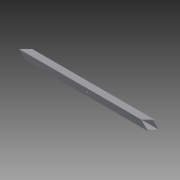
# Autodesk Inventor part: 1x1 support horizontal
Saved by Autodesk Inventor 2015 (Build 190159000, 159)
## iProperties
Created: 2015-01-22
Part Number: 1x1 support horizontal
Material: Generic
Document SubType Name: Modeling
Designer: 215152
Density: 1 g/cm^3
Appearance: Default
Author: 215152
Autodesk Inventor part; units mm, degrees
ref_plane "YZ Plane" through (0, 0, 0) normal (1, 0, 0) x (0, 1, 0)
ref_plane "XZ Plane" through (0, 0, 0) normal (0, 1, 0) x (-1, 0, 0)
ref_plane "XY Plane" through (0, 0, 0) normal (0, 0, 1) x (1, 0, 0)
sketch "Sketch1" plane through (0, 0, 0) normal (1, 0, 0) x (0, 1, 0)
  line L0 (0, 0) -> (-25.4, 0)
  line L1 (-25.4, 0) -> (-25.4, 25.4)
  line L2 (-25.4, 25.4) -> (0, 25.4)
  line L3 (0, 25.4) -> (0, 0)
  line L4 (-3.175, 3.175) -> (-22.225, 3.175)
  line L5 (-22.225, 3.175) -> (-22.225, 22.225)
  line L6 (-22.225, 22.225) -> (-3.175, 22.225)
  line L7 (-3.175, 22.225) -> (-3.175, 3.175)
  dimension "d0" = 25.4
  dimension "d1" = 25.4
  dimension "d2" = 19.05
  dimension "d3" = 19.05
  dimension "d4" = 3.175
  dimension "d5" = 3.175
  constraints: 16 end point, 4 parallel, 2 horizontal, 2 perpendicular
  measures "d0" distance of L1.end L2.end
  measures "d1" distance of L0.end L1.end
  measures "d2" distance of L5.end L6.end
  measures "d3" distance of L4.end L5.end
  measures "d4" distance between parallel lines of L0 L4
  measures "d5" distance between parallel lines of L3 L7
extrude "Extrusion1" add sketch "Sketch1" along normal blind 603.25
sketch "Sketch2" plane through (0, -25.4, 25.4) normal (0, 0, 1) x (1, 0, 0)
  line L0 (0, 0) -> (0, 25.4) projected
  line L1 (0, 0) -> (603.25, 0) projected
  line L2 (603.25, 25.4) -> (603.25, 0) projected
  line L3 (0, 25.4) -> (603.25, 25.4) projected
  point P0 (12.7, 12.7)
  point P1 (301.625, 12.7)
  point P2 (590.55, 12.7)
  dimension "d8" = 12.7
  dimension "d9" = 12.7
  dimension "d10" = 12.7
  dimension "d11" = 12.7
  dimension "d12" = 12.7
  dimension "d13" = 301.625
  measures "d8" distance from line of L0 point (12.7, 12.7)
  measures "d9" distance from line of L1 point (12.7, 12.7)
  measures "d10" distance from line of L1 point (301.625, 12.7)
  measures "d11" distance from line of L1 point (590.55, 12.7)
  measures "d12" distance from line of L2 point (590.55, 12.7)
  measures "d13" distance from line of point (301.625, 12.7) L0
hole "Hole1" at (12.7, -12.7, 25.4) at (301.625, -12.7, 25.4) at (590.55, -12.7, 25.4) direction (0, 0, -1) diameter 6.35 end through all
sketch "Sketch3" plane through (0, -25.4, 0) normal (0, 0, -1) x (-1, 0, 0)
  circle A0 centre (-301.625, 12.7) radius 3.175 projected
  circle A1 centre (-12.7, 12.7) radius 3.175 projected
  circle A2 centre (-590.55, 12.7) radius 3.175 projected
  line L0 (0, 25.4) -> (0, 0) projected
  line L1 (0, 25.4) -> (-603.25, 25.4) projected
  line L2 (-603.25, 0) -> (-603.25, 25.4) projected
  line L3 (0, 0) -> (-603.25, 0) projected
  circle A3 centre (-12.7, 12.7) radius 3.175 projected
  circle A4 centre (-12.7, 12.7) radius 7.9375
  circle A5 centre (-301.625, 12.7) radius 7.9375
  circle A6 centre (-590.55, 12.7) radius 3.175 projected
  circle A7 centre (-590.55, 12.7) radius 7.9375
  dimension "d21" = 15.875
  dimension "d22" = 15.875
  dimension "d23" = 15.875
  constraints: 3 centre point, 3 coincident
  measures "d21" diameter of A4
  measures "d22" diameter of A5
  measures "d23" diameter of A7
extrude "Extrusion2" cut sketch "Sketch3" against normal blind 12.7 contours A4 | A5 | A7
sketch "Sketch4" plane through (0, -25.4, 25.4) normal (0, 0, 1) x (1, 0, 0)
  circle A0 centre (301.625, 12.7) radius 3.175 projected
  circle A1 centre (12.7, 12.7) radius 3.175 projected
  circle A2 centre (590.55, 12.7) radius 3.175 projected
  line L0 (0, 0) -> (0, 25.4) projected
  line L1 (0, 0) -> (603.25, 0) projected
  line L2 (603.25, 25.4) -> (603.25, 0) projected
  line L3 (0, 25.4) -> (603.25, 25.4) projected
  point P0 (38.1, 12.7)
  point P1 (565.15, 12.7)
  dimension "d26" = 12.7
  dimension "d27" = 38.1
  dimension "d28" = 12.7
  dimension "d29" = 38.1
  measures "d26" distance from line of L1 point (38.1, 12.7)
  measures "d27" distance from line of L0 point (38.1, 12.7)
  measures "d28" distance from line of L1 point (565.15, 12.7)
  measures "d29" distance from line of L2 point (565.15, 12.7)
hole "Hole2" at (38.1, -12.7, 25.4) at (565.15, -12.7, 25.4) direction (0, 0, -1) diameter 6.35 end through all
body "Solid1"
